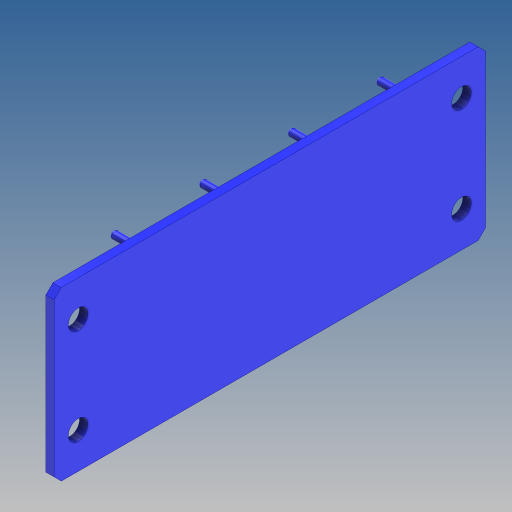
# Autodesk Inventor part: Halterung Gläser1,0
Saved by Autodesk Inventor 2023.3 (Build 273359000, 359)
## iProperties
Created: 2021-10-11
Part Number: Halterung Gläser1,0
Material: Generisch
Document SubType Name: Modeling
Designer: bhelg
Density: 1 g/cm^3
Appearance: Blau - Wandfarbe - glänzend
Author: bhelg
Autodesk Inventor part; units mm, degrees
ref_plane "YZ Plane" through (0, 0, 0) normal (1, 0, 0) x (0, 1, 0)
ref_plane "XZ Plane" through (0, 0, 0) normal (0, 1, 0) x (-1, 0, 0)
ref_plane "XY Plane" through (0, 0, 0) normal (0, 0, 1) x (1, 0, 0)
sketch "Skizze1" plane through (0, 0, 0) normal (0, 1, 0) x (-1, 0, 0)
  line L0 (10.8901, 21.3821) -> (14.3901, 21.3821)
  line L1 (14.3901, 21.3821) -> (14.3901, -158.6179)
  line L2 (14.3901, -158.6179) -> (10.8901, -158.6179)
  line L3 (10.8901, -158.6179) -> (10.8901, 21.3821)
  dimension "d0" = 180
  dimension "d1" = 3.5
  constraints: 8 end point, 3 perpendicular, 1 horizontal
  measures "d0" distance of L0.end L1.end
  measures "d1" distance of L0.start L0.end
extrude "Extrusion1" add sketch "Skizze1" along normal blind 70
sketch "Skizze2" plane through (-14.3901, 0, -158.6179) normal (-1, 0, 0) x (0, 0, 1)
  line L0 (0, 0) -> (180, 0) projected
  circle A0 centre (33, 18) radius 13.7 construction
  circle A1 centre (33, 52) radius 13.7 construction
  circle A2 centre (90, 30) radius 72.5 construction
  line L1 (0, 0) -> (0, 70) projected
  line L2 (0, 70) -> (180, 70) projected
  circle A3 centre (71, 18) radius 13.7 construction
  circle A4 centre (109, 18) radius 13.7 construction
  circle A5 centre (147, 18) radius 13.7 construction
  circle A6 centre (72.7786, 43.5) radius 13.7 construction
  circle A7 centre (109.0755, 43.5) radius 13.7 construction
  circle A8 centre (144.3092, 43.5) radius 13.7 construction
  circle A9 centre (33, 18) radius 15.2
  circle A10 centre (17.8, 18) radius 1.5
  circle A11 centre (33, 33.2) radius 1.5
  circle A12 centre (48.2, 18) radius 1.5
  circle A13 centre (33, 2.8) radius 1.5
  circle A14 centre (33, 52) radius 15.2
  circle A15 centre (17.8, 52) radius 1.5
  circle A16 centre (33, 67.2) radius 1.5
  circle A17 centre (48.2, 52) radius 1.5
  circle A18 centre (33, 36.8) radius 1.5
  circle A19 centre (33, 18) radius 15.7
  circle A20 centre (33, 52) radius 15.7
  point P0 (158.6179, 0)
  dimension "d38" = 27.4
  dimension "d39" = 27.4
  dimension "d42" = 145
  dimension "d43" = 90
  dimension "d44" = 30
  dimension "d50" = 33
  dimension "d51" = 33
  dimension "d52" = 18
  dimension "d53" = 18
  dimension "d63" = 27.4
  dimension "d64" = 27.4
  dimension "d65" = 27.4
  dimension "d66" = 27.4
  dimension "d67" = 27.4
  dimension "d68" = 27.4
  dimension "d69" = 38
  dimension "d70" = 38
  dimension "d71" = 38
  dimension "d98" = 30.4
  dimension "d99" = 3
  dimension "d100" = 3
  dimension "d101" = 3
  dimension "d102" = 3
  dimension "d103" = 30.4
  dimension "d104" = 3
  dimension "d105" = 3
  dimension "d106" = 3
  dimension "d107" = 3
  dimension "d114" = 31.4
  dimension "d115" = 31.4
  constraints: 21 centre point, 8 point on circle, 4 coincident
  measures "d38" diameter of A0
  measures "d39" diameter of A1
  measures "d42" diameter of A2
  measures "d43" horizontal distance of A2.centre L0.start
  measures "d44" vertical distance of L0.start A2.centre
  measures "d50" distance from line of L1 A0.centre
  measures "d51" distance from line of L1 A1.centre
  measures "d52" distance from line of L0 A0.centre
  measures "d53" distance from line of L2 A1.centre
  measures "d63" diameter of A3
  measures "d64" diameter of A4
  measures "d65" diameter of A5
  measures "d66" diameter of A6
  measures "d67" diameter of A7
  measures "d68" diameter of A8
  measures "d69" distance of A3.centre A0.centre
  measures "d70" distance of A4.centre A3.centre
  measures "d71" distance of A4.centre A5.centre
  measures "d98" diameter of A9
  measures "d99" diameter of A10
  measures "d100" diameter of A11
  measures "d101" diameter of A12
  measures "d102" diameter of A13
  measures "d103" diameter of A14
  measures "d104" diameter of A15
  measures "d105" diameter of A16
  measures "d106" diameter of A17
  measures "d107" diameter of A18
  measures "d114" diameter of A19
  measures "d115" diameter of A20
sketch "Skizze3" plane through (-14.3901, 0, -158.6179) normal (-1, 0, 0) x (0, 0, 1)
  line L0 (0, 0) -> (180, 0) projected
  line L1 (0, 70) -> (180, 70) projected
  line L2 (180, 0) -> (180, 70) projected
  line L3 (0, 0) -> (0, 70) projected
  line L4 (170, 15) -> (170, 55)
  line L5 (10, 15) -> (10, 55)
  point P0 (158.6179, 0)
  dimension "d83" = 40
  dimension "d84" = 40
  dimension "d85" = 15
  dimension "d87" = 15
  dimension "d88" = 15
  dimension "d89" = 10
  dimension "d90" = 10
  dimension "d160" = 70
  dimension "d161" = 70
  dimension "d162" = 160
  constraints: 4 end point, 2 vertical
  measures "d83" distance of L5.end L5.start
  measures "d84" distance of L4.end L4.start
  measures "d85" distance from line of L0 L4.start
  measures "d87" distance from line of L0 L5.start
  measures "d88" distance from line of L1 L5.end
  measures "d89" distance from line of L2 L4.start
  measures "d90" distance from line of L3 L5.start
  measures "d160" distance of L0.end L1.end
  measures "d161" distance of L0.start L1.start
  measures "d162" distance of L4.start L5.start
hole "Bohrung1" at (-14.3901, 15, -148.6179) at (-14.3901, 55, -148.6179) at (-14.3901, 15, 11.3821) at (-14.3901, 55, 11.3821) direction (1, 0, 0) diameter 8.2 end through all
extrude "Extrusion3" add sketch "Skizze2" along normal blind 8 contours A9 A12 | A9 A12 A19 | A11 A9 | A9 A11 A19 | A12 A19 | A13 A19 A9 | A9 A13 | A19 A11 | A13 A19 | A10 A9 | A9 A10 A19 | A19 A10 | A14 A17 | A14 A17 A20 | A16 A14 | A14 A16 A20 | A17 A20 | A18 A20 A14 | A14 A18 | A20 A16 | A18 A20 | A15 A14 | A14 A15 A20 | A20 A15
pattern_linear "Rechteckige Anordnung2" count 4 spacing 37 along (0, 0, 1) of "Extrusion3"
fillet "Rundung1" radius 1 32 edges at (-22.3901, 2.8, -127.1179) (-22.3901, 18, -142.3179) (-22.3901, 18, -111.9179) (-22.3901, 33.2, -127.1179) (-22.3901, 36.8, -127.1179) (-22.3901, 52, -142.3179) (-22.3901, 52, -111.9179) (-22.3901, 67.2, -127.1179) (-22.3901, 18, -105.3179) (-22.3901, 2.8, -90.1179) (-22.3901, 33.2, -90.1179) (-22.3901, 36.8, -90.1179) (-22.3901, 52, -105.3179) (-22.3901, 18, -74.9179) (-22.3901, 67.2, -90.1179) (-22.3901, 52, -74.9179) (-22.3901, 52, -68.3179) (-22.3901, 36.8, -53.1179) (-22.3901, 33.2, -53.1179) (-22.3901, 18, -68.3179) (-22.3901, 2.8, -53.1179) (-22.3901, 18, -37.9179) (-22.3901, 18, -31.3179) (-22.3901, 2.8, -16.1179) (-22.3901, 18, -0.9179) (-22.3901, 33.2, -16.1179) (-22.3901, 36.8, -16.1179) (-22.3901, 52, -31.3179) (-22.3901, 52, -37.9179) (-22.3901, 67.2, -53.1179) (-22.3901, 67.2, -16.1179) (-22.3901, 52, -0.9179)
sketch "Skizze4" plane through (-14.3901, 0, -158.6179) normal (-1, 0, 0) x (0, 0, 1)
  line L0 (0, 0) -> (180, 0)
  circle A0 centre (33, 18) radius 13.7 construction
  circle A1 centre (33, 52) radius 13.7 construction
  circle A2 centre (90, 30) radius 72.5 construction
  line L1 (0, 0) -> (0, 70)
  line L2 (0, 70) -> (180, 70)
  circle A3 centre (71, 18) radius 13.7 construction
  circle A4 centre (109, 18) radius 13.7 construction
  circle A5 centre (147, 18) radius 13.7 construction
  circle A6 centre (72.7786, 43.5) radius 13.7 construction
  circle A7 centre (109.0755, 43.5) radius 13.7 construction
  circle A8 centre (144.3092, 43.5) radius 13.7 construction
  circle A9 centre (33, 18) radius 15.2
  circle A10 centre (17.8, 18) radius 1.5
  circle A11 centre (33, 33.2) radius 1.5
  circle A12 centre (48.2, 18) radius 1.5
  circle A13 centre (33, 2.8) radius 1.5
  circle A14 centre (33, 52) radius 15.2
  circle A15 centre (17.8, 52) radius 1.5
  circle A16 centre (33, 67.2) radius 1.5
  circle A17 centre (48.2, 52) radius 1.5
  circle A18 centre (33, 36.8) radius 1.5
  circle A19 centre (33, 18) radius 15.7
  circle A20 centre (33, 52) radius 15.7
  point P0 (158.6179, 0)
  point P1 (158.6179, 0)
  point P2 (31.5642, 67.6342)
  point P3 (17.3658, 53.4358)
  point P4 (17.874, 53.4982)
  point P5 (31.5018, 67.126)
  point P6 (17.3658, 50.5642)
  point P7 (31.5642, 36.3658)
  point P8 (31.5018, 36.874)
  point P9 (17.874, 50.5018)
  point P10 (48.6342, 53.4358)
  point P11 (34.4358, 67.6342)
  point P12 (34.4982, 67.126)
  point P13 (48.126, 53.4982)
  point P14 (34.4358, 36.3658)
  point P15 (48.6342, 50.5642)
  point P16 (48.126, 50.5018)
  point P17 (34.4982, 36.874)
  point P18 (34.4358, 2.3658)
  point P19 (48.6342, 16.5642)
  point P20 (48.126, 16.5018)
  point P21 (34.4982, 2.874)
  point P22 (48.6342, 19.4358)
  point P23 (34.4358, 33.6342)
  point P24 (34.4982, 33.126)
  point P25 (48.126, 19.4982)
  point P26 (31.5642, 33.6342)
  point P27 (17.3658, 19.4358)
  point P28 (17.874, 19.4982)
  point P29 (31.5018, 33.126)
  point P30 (17.3658, 16.5642)
  point P31 (31.5642, 2.3658)
  point P32 (31.5018, 2.874)
  point P33 (17.874, 16.5018)
  dimension "d116" = 27.4
  dimension "d117" = 27.4
  dimension "d118" = 145
  dimension "d119" = 90
  dimension "d120" = 30
  dimension "d121" = 33
  dimension "d122" = 33
  dimension "d123" = 18
  dimension "d124" = 18
  dimension "d125" = 27.4
  dimension "d126" = 27.4
  dimension "d127" = 27.4
  dimension "d128" = 27.4
  dimension "d129" = 27.4
  dimension "d130" = 27.4
  dimension "d131" = 38
  dimension "d132" = 38
  dimension "d133" = 38
  dimension "d134" = 30.4
  dimension "d135" = 3
  dimension "d136" = 3
  dimension "d137" = 3
  dimension "d138" = 3
  dimension "d139" = 30.4
  dimension "d140" = 3
  dimension "d141" = 3
  dimension "d142" = 3
  dimension "d143" = 3
  dimension "d144" = 31.4
  dimension "d145" = 31.4
  constraints: 21 centre point, 8 point on circle, 6 end point, 4 coincident
  measures "d116" diameter of A0
  measures "d117" diameter of A1
  measures "d118" diameter of A2
  measures "d119" horizontal distance of A2.centre L0.start
  measures "d120" vertical distance of L0.start A2.centre
  measures "d121" distance from line of L1 A0.centre
  measures "d122" distance from line of L1 A1.centre
  measures "d123" distance from line of L0 A0.centre
  measures "d124" distance from line of L2 A1.centre
  measures "d125" diameter of A3
  measures "d126" diameter of A4
  measures "d127" diameter of A5
  measures "d128" diameter of A6
  measures "d129" diameter of A7
  measures "d130" diameter of A8
  measures "d131" distance of A3.centre A0.centre
  measures "d132" distance of A4.centre A3.centre
  measures "d133" distance of A4.centre A5.centre
  measures "d134" diameter of A9
  measures "d135" diameter of A10
  measures "d136" diameter of A11
  measures "d137" diameter of A12
  measures "d138" diameter of A13
  measures "d139" diameter of A14
  measures "d140" diameter of A15
  measures "d141" diameter of A16
  measures "d142" diameter of A17
  measures "d143" diameter of A18
  measures "d144" diameter of A19
  measures "d145" diameter of A20
extrude "Extrusion4" cut sketch "Skizze4" against normal blind 0.5 contours A9 A11 A19 A12 | A12 A19 A13 A9 | A9 A10 A19 A11 | A13 A19 A10 A9 | A14 A16 A20 A17 | A17 A20 A18 A14 | A14 A15 A20 A16 | A18 A20 A15 A14
pattern_linear "Rechteckige Anordnung3" count 4 spacing 37 along (0, 0, 1) of "Extrusion4"
chamfer "Fase1" distance 3 angle 45 4 edges at (-12.6401, 0, 21.3821) (-12.6401, 70, 21.3821) (-12.6401, 70, -158.6179) (-12.6401, 0, -158.6179)
